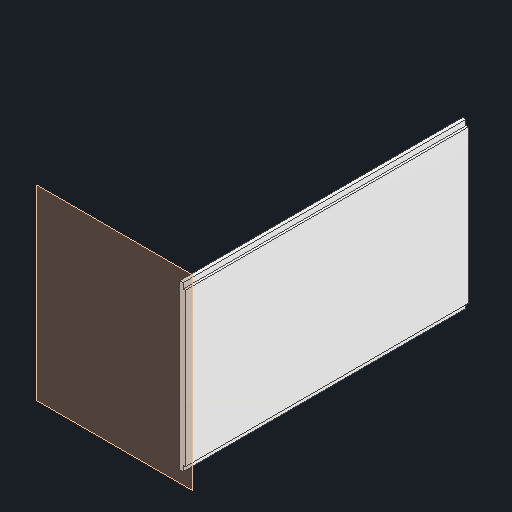
# Autodesk Inventor part: Lid1
Saved by Autodesk Inventor 2026.1 (Build 301233000, 233)
## iProperties
Created: 2025-08-01
Part Number: Lid1
Material: Plastic, Opaque White
Document SubType Name: Sheet Metal
Designer: Cupri
Density: 0.952 g/cm^3
Sheet Metal Rule: Default
Appearance: Smooth - White
Author: Cupri
Autodesk Inventor part; units mm, degrees
ref_plane "YZ Plane" through (0, 0, 0) normal (1, 0, 0) x (0, 1, 0)
ref_plane "XZ Plane" through (0, 0, 0) normal (0, 1, 0) x (-1, 0, 0)
ref_plane "Work Plane1" through (0, 0, 0) normal (0, 0, 1) x (1, 0, 0)
sketch "Sketch1" plane through (0, 0, 0) normal (0, 0, 1) x (1, 0, 0)
  line L0 (62.538, -67.5) -> (62.538, 67.5) projected
  line L1 (57.538, 75) -> (57.538, -75) projected
  line L2 (60.538, 72.3) -> (57.538, 72.3) projected
  line L3 (60.538, 67.5) -> (60.538, 72.5) projected
  line L4 (60.538, -72.3) -> (57.538, -72.3) projected
  line L5 (60.538, -72.5) -> (60.538, -67.5) projected
  line L6 (62.538, -67.5) -> (60.538, -67.5) projected
  line L7 (57.538, 72.3) -> (60.538, 72.3)
  line L8 (60.538, 72.3) -> (60.538, -72.3)
  line L9 (60.538, -72.3) -> (57.538, -72.3)
  line L10 (57.538, -72.3) -> (57.538, 72.3)
  line L11 (62.538, -67.5) -> (60.538, -67.5)
  line L12 (60.538, -67.5) -> (60.538, 67.5)
  line L13 (60.538, 67.5) -> (62.538, 67.5)
  line L14 (62.538, 67.5) -> (62.538, -67.5)
  spline S0 degree 3 poles (88.3509, 80.1315) (86.4042, 80.1549) (83.4825, 80.1842) (78.158, 80.2283) (74.9959, 80.2506) (69.3132, 80.2873) (67.2613, 80.2982) (65.6092, 80.307) knots 0.050298 0.050298 0.050298 0.050298 4.412638 4.412638 8.294204 8.294204 12.536981 12.536981 12.536981 12.536981 projected
  point P0 (0, 0)
  point P1 (62.538, 67.5)
  point P2 (57.538, 72.3)
  point P3 (57.538, -72.3)
  constraints: 16 end point, 4 parallel, 2 horizontal, 2 perpendicular
ref_plane "Work Plane2" through (-62.538, -75, -250) normal (0, 0, 1) x (1, 0, 0)
extrude "Extrusion1" add sketch "Sketch1" against normal up to surface (250 mm away)
equation "\"BendRadius\" = Thickness"
equation "\"BendReliefWidth\" = Thickness"
equation "\"BendReliefDepth\" = 0.5 * Thickness"
equation "\"CornerReliefSize\" = 4 * Thickness"
equation "\"MinimumRemnant\" = 2 * Thickness"
equation "\"TransitionRadius\" = BendRadius"
equation "\"JacobiRadiusSize\" = BendRadius"
equation "\"GapSize\" = Thickness"
equation "\"Thickness\" = 3.048"
body "Solid1"
